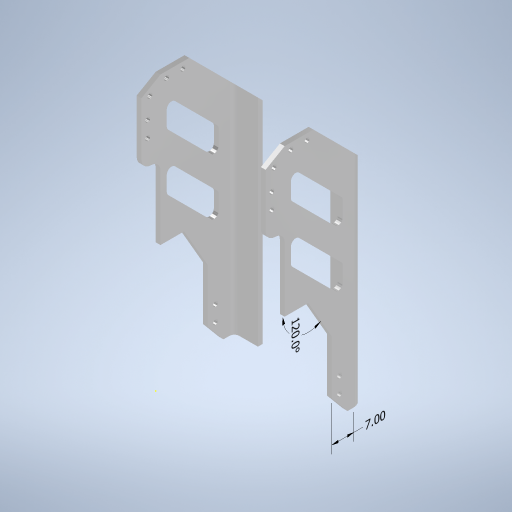
# Autodesk Inventor part: side
Saved by Autodesk Inventor 2024.1 (Build 281209000, 209)
## iProperties
Created: 2024-10-11
Part Number: side
Material: アルミニウム 6061
Document SubType Name: Sheet Metal
Designer: hibik
Density: 2.7 g/cm^3
Sheet Metal Rule: Default_mm
Appearance: アルミニウム - フラット
Author: hibik
Autodesk Inventor part; units mm, degrees
ref_plane "YZ Plane" through (0, 0, 0) normal (1, 0, 0) x (0, 1, 0)
ref_plane "XZ Plane" through (0, 0, 0) normal (0, 1, 0) x (-1, 0, 0)
ref_plane "XY Plane" through (0, 0, 0) normal (0, 0, 1) x (1, 0, 0)
sketch "スケッチ1" plane through (0, 0, 0) normal (1, 0, 0) x (0, 1, 0)
  line L0 (0, 0) -> (85, 0)
  line L1 (85, 0) -> (85, -20)
  line L2 (85, -20) -> (0, -20)
  line L3 (0, -20) -> (0, 0)
  circle A0 centre (0, -20) radius 1.6
  line L4 (-4, 0) -> (85, 0)
  line L5 (85, 0) -> (85, -25)
  line L6 (85, -25) -> (-4, -25)
  line L7 (-4, -25) -> (-4, 0)
  line L8 (-23, 0) -> (103, 0)
  line L9 (11, 0) -> (11, -15)
  line L10 (11, -15) -> (-0.9175, -25)
  line L11 (11, -15) -> (28.0096, -15)
  line L12 (28.0096, -15) -> (41, -7.5)
  line L13 (41, -7.5) -> (41, 0)
  circle A1 centre (0, -20) radius 5
  point P0 (4.9999, -20.0347)
  point P1 (0, -25)
  dimension "d0" = 85
  dimension "d1" = 20
  dimension "d2" = 3.2
  dimension "d3" = 4
  dimension "d4" = 5
  dimension "d5" = 5
  dimension "d6" = 11
  dimension "d7" = 50
  dimension "d8" = 7.5
  dimension "d9" = 120
  dimension "d10" = 41
  dimension "d11" = 15
  dimension "d12" = 10
  measures "d0" distance of L1.end L2.end
  measures "d1" distance of L2.end L0.start
  measures "d2" diameter of A0
  measures "d3" distance between parallel lines of L3 L7
  measures "d4" distance between parallel lines of L6 L2
  measures "d5" vertical distance of L9.end L2.end
  measures "d6" distance from line of L9 A0.centre
  measures "d7" angle of L9 L10
  measures "d8" distance of L12.end L13.end
  measures "d9" angle of L12 L13
  measures "d10" distance from line of L2.end L13
  measures "d11" distance between parallel lines of L0 L11
  measures "d12" diameter of A1
extrude "プレート1" add sketch "スケッチ1" along normal blind 1.5 contours L0 L1 L2 L10 L11 L12 L13 | L2 L5 L6 A1 L10
sketch "スケッチ2" plane through (1.5, 0, 0) normal (1, 0, 0) x (0, 0, -1)
  line L0 (2, 85) -> (2, 41)
  line L1 (0, 41) -> (0, 85) projected
  line L2 (7.5, 41) -> (0, 41) projected
  line L3 (0, 85) -> (25, 85) projected
  line L4 (2, 81) -> (18.5, 64.5)
  line L5 (18.5, 64.5) -> (18.5, 55.5)
  line L6 (18.5, 55.5) -> (2, 72)
  line L7 (2, 63) -> (18.5, 46.5)
  line L8 (18.5, 46.5) -> (18.5, 37.5)
  line L9 (18.5, 37.5) -> (2, 54)
  line L10 (25, 85) -> (25, 0) projected
  point P0 (0, 0)
  dimension "d14" = 2
  dimension "d15" = 135
  dimension "d16" = 9
  dimension "d17" = 6.5
  dimension "d18" = 9
  dimension "d19" = 13
  constraints: 14 end point, 5 point on line, 4 equal length, 2 collinear, 1 midpoint, 1 vertical
  measures "d14" distance between parallel lines of L1 L0
  measures "d15" angle of L0 L6
  measures "d16" distance of L4.end L5.end
  measures "d17" distance between parallel lines of L10 L5
  measures "d18" distance of L7.start L6.end
  measures "d19" distance from line of L2 L9.end
extrude "切り取り1" cut sketch "スケッチ2" against normal blind 1.5 contours L4 L5 L6 L0 | L7 L8 L9 L0
sketch "スケッチ3" plane through (1.5, 0, -23.5) normal (0, 0, -1) x (-1, 0, 0)
  line L0 (0, 85) -> (0, 0)
  line L1 (0, 0) -> (41, 0)
  line L2 (41, 0) -> (41, 85)
  line L3 (41, 85) -> (0, 85)
  constraints: 6 end point, 1 horizontal, 1 perpendicular, 1 vertical
edge flange "フランジ1" height 41 angle 90 thickness 1.5 bend radius 1.5 thickness toward (0, 0, -1) relief straight relief width 1.5 relief depth 0.75 edges at (0, 42.5, -25) wall of the first edge with corners at (1.5, 85, -23.5) (1.5, 0, -23.5) (-39.5, 0, -23.5) (-39.5, 85, -23.5)
bend "曲げ1"
corner "コーナー1"
sketch "スケッチ4" plane through (-38, 0, -25) normal (-1, 0, 0) x (0, -1, 0)
  line L0 (-85, 0) -> (0, 0)
  line L1 (0, 0) -> (0, 25)
  line L2 (0, 25) -> (-85, 25)
  line L3 (-85, 25) -> (-85, 0)
  constraints: 6 end point, 1 horizontal, 1 perpendicular, 1 vertical
edge flange "フランジ2" height 25 angle 90 thickness 1.5 bend radius 1.5 thickness toward (-1, 0, 0) relief straight relief width 1.5 relief depth 0.75 edges at (-39.5, 42.5, -23.5) wall of the first edge with corners at (-38, 85, -25) (-38, 0, -25) (-38, 0, 0) (-38, 85, 0)
bend "曲げ2"
corner "コーナー2"
sketch "スケッチ5" plane through (-38, 0, 0) normal (1, 0, 0) x (0, 0, -1)
  line L0 (22, 4.5826) -> (22, 85) projected
  line L1 (0, 85) -> (22, 85) projected
  line L2 (7.5, 41) -> (0, 41) projected
  line L3 (15, 28.0096) -> (7.5, 41) projected
  line L4 (15, 11) -> (15, 28.0096) projected
  line L5 (20.0347, 4.9999) -> (15, 11) projected
  arc A0 (22, 4.5826) -> (20.0347, 4.9999) centre (20, 0) ccw projected
  line L6 (18.5, 37.5) -> (2, 54) projected
  line L7 (2, 54) -> (2, 63) projected
  line L8 (2, 63) -> (18.5, 46.5) projected
  line L9 (18.5, 46.5) -> (18.5, 37.5) projected
  line L10 (2, 72) -> (2, 81) projected
  line L11 (22, 0) -> (22, 85) projected
  line L12 (22, 85) -> (0, 85) projected
  line L13 (0, 85) -> (0, 0) projected
  line L14 (22, 0) -> (0, 0) projected
  line L15 (2, 81) -> (18.5, 64.5) projected
  line L16 (18.5, 64.5) -> (18.5, 55.5) projected
  line L17 (18.5, 55.5) -> (2, 72) projected
  line L18 (0, 41) -> (0, 85) projected
  point P0 (0, 0)
  point P1 (0, 41)
  point P2 (22, 4.5826)
  point P3 (2, 85)
extrude "押し出し1" cut sketch "スケッチ5" against normal through all contours L11 L14 L13 L2 L3 L4 L5 A0 | L6 L7 L8 L9 | L10 L15 L16 L17
sketch "スケッチ7" plane through (-1.5, 0, -25) normal (0, 0, -1) x (-1, 0, 0)
  line L0 (0, 85) -> (35, 85) projected
  line L1 (6, 85) -> (29, 85)
  line L2 (29, 85) -> (29, 0)
  line L3 (29, 0) -> (6, 0)
  line L4 (6, 0) -> (6, 85)
  line L5 (0, 85) -> (0, 0) projected
  line L6 (35, 0) -> (35, 85) projected
  line L7 (6.1906, 67) -> (15.1906, 67) construction
  line L8 (15.1906, 67) -> (10.6906, 59.2058) construction
  line L9 (10.6906, 59.2058) -> (6.1906, 67) construction
  arc A0 (8.7887, 67) -> (7.4896, 64.75) centre (8.7887, 65.5) ccw
  arc A1 (13.8916, 64.75) -> (12.5925, 67) centre (12.5925, 65.5) ccw
  arc A2 (9.3916, 61.4558) -> (11.9896, 61.4558) centre (10.6906, 62.2058) ccw
  line L10 (17.5, 67) -> (13, 59.2058) construction
  line L11 (13, 59.2058) -> (22, 59.2058) construction
  line L12 (22, 59.2058) -> (17.5, 67) construction
  arc A3 (18.799, 64.75) -> (16.201, 64.75) centre (17.5, 64) ccw
  arc A4 (14.299, 61.4558) -> (15.5981, 59.2058) centre (15.5981, 60.7058) ccw
  arc A5 (19.4019, 59.2058) -> (20.701, 61.4558) centre (19.4019, 60.7058) ccw
  line L13 (8.7887, 67) -> (12.5925, 67)
  line L14 (13.8916, 64.75) -> (11.9896, 61.4558)
  line L15 (7.4896, 64.75) -> (9.3916, 61.4558)
  line L16 (16.201, 64.75) -> (14.299, 61.4558)
  line L17 (15.5981, 59.2058) -> (19.4019, 59.2058)
  line L18 (20.701, 61.4558) -> (18.799, 64.75)
  line L19 (19.8094, 67) -> (28.8094, 67) construction
  line L20 (28.8094, 67) -> (24.3094, 59.2058) construction
  line L21 (24.3094, 59.2058) -> (19.8094, 67) construction
  arc A6 (22.4075, 67) -> (21.1084, 64.75) centre (22.4075, 65.5) ccw
  arc A7 (27.5104, 64.75) -> (26.2113, 67) centre (26.2113, 65.5) ccw
  arc A8 (23.0104, 61.4558) -> (25.6084, 61.4558) centre (24.3094, 62.2058) ccw
  line L22 (22.4075, 67) -> (26.2113, 67)
  line L23 (27.5104, 64.75) -> (25.6084, 61.4558)
  line L24 (21.1084, 64.75) -> (23.0104, 61.4558)
  line L25 (6, 58.2058) -> (29, 58.2058) construction
  line L26 (6.1906, 49.4115) -> (15.1906, 49.4115) construction
  line L27 (15.1906, 49.4115) -> (10.6906, 57.2058) construction
  line L28 (10.6906, 57.2058) -> (6.1906, 49.4115) construction
  arc A9 (7.4896, 51.6615) -> (8.7887, 49.4115) centre (8.7887, 50.9115) ccw
  arc A10 (12.5925, 49.4115) -> (13.8916, 51.6615) centre (12.5925, 50.9115) ccw
  arc A11 (11.9896, 54.9558) -> (9.3916, 54.9558) centre (10.6906, 54.2058) ccw
  line L29 (17.5, 49.4115) -> (13, 57.2058) construction
  line L30 (13, 57.2058) -> (22, 57.2058) construction
  line L31 (22, 57.2058) -> (17.5, 49.4115) construction
  arc A12 (16.201, 51.6615) -> (18.799, 51.6615) centre (17.5, 52.4115) ccw
  arc A13 (15.5981, 57.2058) -> (14.299, 54.9558) centre (15.5981, 55.7058) ccw
  arc A14 (20.701, 54.9558) -> (19.4019, 57.2058) centre (19.4019, 55.7058) ccw
  line L32 (8.7887, 49.4115) -> (12.5925, 49.4115)
  line L33 (13.8916, 51.6615) -> (11.9896, 54.9558)
  line L34 (7.4896, 51.6615) -> (9.3916, 54.9558)
  line L35 (16.201, 51.6615) -> (14.299, 54.9558)
  line L36 (15.5981, 57.2058) -> (19.4019, 57.2058)
  line L37 (20.701, 54.9558) -> (18.799, 51.6615)
  line L38 (19.8094, 49.4115) -> (28.8094, 49.4115) construction
  line L39 (28.8094, 49.4115) -> (24.3094, 57.2058) construction
  line L40 (24.3094, 57.2058) -> (19.8094, 49.4115) construction
  arc A15 (21.1084, 51.6615) -> (22.4075, 49.4115) centre (22.4075, 50.9115) ccw
  arc A16 (26.2113, 49.4115) -> (27.5104, 51.6615) centre (26.2113, 50.9115) ccw
  line L41 (27.5104, 51.6615) -> (25.6084, 54.9558)
  arc A17 (25.6084, 54.9558) -> (23.0104, 54.9558) centre (24.3094, 54.2058) ccw
  line L42 (22.4075, 49.4115) -> (26.2113, 49.4115)
  line L43 (21.1084, 51.6615) -> (23.0104, 54.9558)
  arc A18 (5.1802, 64.75) -> (2.5822, 64.75) centre (3.8812, 64) ccw
  arc A19 (5.7831, 59.2058) -> (7.0822, 61.4558) centre (5.7831, 60.7058) ccw
  line L44 (7.0822, 61.4558) -> (5.1802, 64.75)
  line L45 (5.7831, 59.2058) -> (-10.927, 59.2058)
  arc A20 (32.4178, 64.75) -> (29.8198, 64.75) centre (31.1188, 64) ccw
  arc A21 (27.9178, 61.4558) -> (29.2169, 59.2058) centre (29.2169, 60.7058) ccw
  line L46 (29.8198, 64.75) -> (27.9178, 61.4558)
  line L47 (29.2169, 59.2058) -> (29, 59.2058)
  line L48 (7.0822, 54.9558) -> (5.1802, 51.6615)
  arc A22 (2.5822, 51.6615) -> (5.1802, 51.6615) centre (3.8812, 52.4115) ccw
  arc A23 (7.0822, 54.9558) -> (5.7831, 57.2058) centre (5.7831, 55.7058) ccw
  line L49 (5.7831, 57.2058) -> (-10.927, 57.2058)
  line L50 (29.8198, 51.6615) -> (27.9178, 54.9558)
  arc A24 (29.8198, 51.6615) -> (32.4178, 51.6615) centre (31.1188, 52.4115) ccw
  arc A25 (29.2169, 57.2058) -> (27.9178, 54.9558) centre (29.2169, 55.7058) ccw
  line L51 (29.2169, 57.2058) -> (29, 57.2058)
  line L52 (6.1906, 47.4115) -> (15.1906, 47.4115) construction
  line L53 (15.1906, 47.4115) -> (10.6906, 39.6173) construction
  arc A26 (9.3916, 41.8673) -> (11.9896, 41.8673) centre (10.6906, 42.6173) ccw
  line L54 (8.7887, 47.4115) -> (12.5925, 47.4115)
  line L55 (13.8916, 45.1615) -> (11.9896, 41.8673)
  arc A27 (13.8916, 45.1615) -> (12.5925, 47.4115) centre (12.5925, 45.9115) ccw
  arc A28 (14.299, 41.8673) -> (15.5981, 39.6173) centre (15.5981, 41.1173) ccw
  line L56 (16.201, 45.1615) -> (14.299, 41.8673)
  arc A29 (18.799, 45.1615) -> (16.201, 45.1615) centre (17.5, 44.4115) ccw
  line L57 (17.5, 47.4115) -> (13, 39.6173) construction
  arc A30 (27.9178, 41.8673) -> (29.2169, 39.6173) centre (29.2169, 41.1173) ccw
  line L58 (29.8198, 45.1615) -> (27.9178, 41.8673)
  arc A31 (32.4178, 45.1615) -> (29.8198, 45.1615) centre (31.1188, 44.4115) ccw
  line L59 (29.2169, 39.6173) -> (29, 39.6173)
  line L60 (22, 39.6173) -> (17.5, 47.4115) construction
  arc A32 (19.4019, 39.6173) -> (20.701, 41.8673) centre (19.4019, 41.1173) ccw
  line L61 (27.5104, 45.1615) -> (25.6084, 41.8673)
  arc A33 (23.0104, 41.8673) -> (25.6084, 41.8673) centre (24.3094, 42.6173) ccw
  arc A34 (27.5104, 45.1615) -> (26.2113, 47.4115) centre (26.2113, 45.9115) ccw
  line L62 (28.8094, 47.4115) -> (24.3094, 39.6173) construction
  line L63 (22.4075, 47.4115) -> (26.2113, 47.4115)
  line L64 (19.8094, 47.4115) -> (28.8094, 47.4115) construction
  line L65 (21.1084, 45.1615) -> (23.0104, 41.8673)
  line L66 (24.3094, 39.6173) -> (19.8094, 47.4115) construction
  line L67 (20.701, 41.8673) -> (18.799, 45.1615)
  arc A35 (22.4075, 47.4115) -> (21.1084, 45.1615) centre (22.4075, 45.9115) ccw
  arc A36 (20.701, 35.3673) -> (19.4019, 37.6173) centre (19.4019, 36.1173) ccw
  line L68 (20.701, 35.3673) -> (18.799, 32.0731)
  line L69 (22, 37.6173) -> (17.5, 29.8231) construction
  arc A37 (16.201, 32.0731) -> (18.799, 32.0731) centre (17.5, 32.8231) ccw
  line L70 (15.5981, 37.6173) -> (19.4019, 37.6173)
  line L71 (13, 37.6173) -> (22, 37.6173) construction
  line L72 (16.201, 32.0731) -> (14.299, 35.3673)
  line L73 (17.5, 29.8231) -> (13, 37.6173) construction
  arc A38 (15.5981, 37.6173) -> (14.299, 35.3673) centre (15.5981, 36.1173) ccw
  line L74 (6.1906, 29.8231) -> (15.1906, 29.8231) construction
  line L75 (15.1906, 29.8231) -> (10.6906, 37.6173) construction
  line L76 (10.6906, 37.6173) -> (6.1906, 29.8231) construction
  arc A39 (7.4896, 32.0731) -> (8.7887, 29.8231) centre (8.7887, 31.3231) ccw
  line L77 (5.7831, 37.6173) -> (-10.927, 37.6173)
  arc A40 (7.0822, 35.3673) -> (5.7831, 37.6173) centre (5.7831, 36.1173) ccw
  arc A41 (2.5822, 32.0731) -> (5.1802, 32.0731) centre (3.8812, 32.8231) ccw
  line L78 (7.0822, 35.3673) -> (5.1802, 32.0731)
  arc A42 (11.9896, 35.3673) -> (9.3916, 35.3673) centre (10.6906, 34.6173) ccw
  line L79 (7.4896, 32.0731) -> (9.3916, 35.3673)
  line L80 (13.8916, 32.0731) -> (11.9896, 35.3673)
  line L81 (8.7887, 29.8231) -> (12.5925, 29.8231)
  arc A43 (12.5925, 29.8231) -> (13.8916, 32.0731) centre (12.5925, 31.3231) ccw
  line L82 (13, 39.6173) -> (22, 39.6173) construction
  line L83 (15.5981, 39.6173) -> (19.4019, 39.6173)
  line L84 (6, 38.6173) -> (29, 38.6173) construction
  line L85 (27.5104, 32.0731) -> (25.6084, 35.3673)
  line L86 (28.8094, 29.8231) -> (24.3094, 37.6173) construction
  arc A44 (26.2113, 29.8231) -> (27.5104, 32.0731) centre (26.2113, 31.3231) ccw
  arc A45 (25.6084, 35.3673) -> (23.0104, 35.3673) centre (24.3094, 34.6173) ccw
  line L87 (21.1084, 32.0731) -> (23.0104, 35.3673)
  arc A46 (21.1084, 32.0731) -> (22.4075, 29.8231) centre (22.4075, 31.3231) ccw
  line L88 (24.3094, 37.6173) -> (19.8094, 29.8231) construction
  line L89 (22.4075, 29.8231) -> (26.2113, 29.8231)
  arc A47 (29.2169, 37.6173) -> (27.9178, 35.3673) centre (29.2169, 36.1173) ccw
  line L90 (19.8094, 29.8231) -> (28.8094, 29.8231) construction
  line L91 (29.8198, 32.0731) -> (27.9178, 35.3673)
  line L92 (29.2169, 37.6173) -> (29, 37.6173)
  arc A48 (29.8198, 32.0731) -> (32.4178, 32.0731) centre (31.1188, 32.8231) ccw
  line L93 (10.6906, 39.6173) -> (6.1906, 47.4115) construction
  arc A49 (8.7887, 47.4115) -> (7.4896, 45.1615) centre (8.7887, 45.9115) ccw
  line L94 (7.4896, 45.1615) -> (9.3916, 41.8673)
  arc A50 (5.7831, 39.6173) -> (7.0822, 41.8673) centre (5.7831, 41.1173) ccw
  line L95 (7.0822, 41.8673) -> (5.1802, 45.1615)
  arc A51 (5.1802, 45.1615) -> (2.5822, 45.1615) centre (3.8812, 44.4115) ccw
  line L96 (5.7831, 39.6173) -> (-10.927, 39.6173)
  line L97 (6.1906, 27.8231) -> (15.1906, 27.8231) construction
  line L98 (15.1906, 27.8231) -> (10.6906, 20.0289) construction
  arc A52 (9.3916, 22.2789) -> (11.9896, 22.2789) centre (10.6906, 23.0289) ccw
  line L99 (8.7887, 27.8231) -> (12.5925, 27.8231)
  line L100 (13.8916, 25.5731) -> (11.9896, 22.2789)
  arc A53 (13.8916, 25.5731) -> (12.5925, 27.8231) centre (12.5925, 26.3231) ccw
  arc A54 (14.299, 22.2789) -> (15.5981, 20.0289) centre (15.5981, 21.5289) ccw
  line L101 (16.201, 25.5731) -> (14.299, 22.2789)
  arc A55 (18.799, 25.5731) -> (16.201, 25.5731) centre (17.5, 24.8231) ccw
  line L102 (17.5, 27.8231) -> (13, 20.0289) construction
  arc A56 (27.9178, 22.2789) -> (29.2169, 20.0289) centre (29.2169, 21.5289) ccw
  line L103 (29.8198, 25.5731) -> (27.9178, 22.2789)
  arc A57 (32.4178, 25.5731) -> (29.8198, 25.5731) centre (31.1188, 24.8231) ccw
  line L104 (29.2169, 20.0289) -> (29, 20.0289)
  line L105 (22, 20.0289) -> (17.5, 27.8231) construction
  arc A58 (19.4019, 20.0289) -> (20.701, 22.2789) centre (19.4019, 21.5289) ccw
  line L106 (27.5104, 25.5731) -> (25.6084, 22.2789)
  arc A59 (23.0104, 22.2789) -> (25.6084, 22.2789) centre (24.3094, 23.0289) ccw
  arc A60 (27.5104, 25.5731) -> (26.2113, 27.8231) centre (26.2113, 26.3231) ccw
  line L107 (28.8094, 27.8231) -> (24.3094, 20.0289) construction
  line L108 (22.4075, 27.8231) -> (26.2113, 27.8231)
  line L109 (19.8094, 27.8231) -> (28.8094, 27.8231) construction
  line L110 (21.1084, 25.5731) -> (23.0104, 22.2789)
  line L111 (24.3094, 20.0289) -> (19.8094, 27.8231) construction
  line L112 (20.701, 22.2789) -> (18.799, 25.5731)
  arc A61 (22.4075, 27.8231) -> (21.1084, 25.5731) centre (22.4075, 26.3231) ccw
  arc A62 (20.701, 15.7789) -> (19.4019, 18.0289) centre (19.4019, 16.5289) ccw
  line L113 (20.701, 15.7789) -> (18.799, 12.4846)
  line L114 (22, 18.0289) -> (17.5, 10.2346) construction
  arc A63 (16.201, 12.4846) -> (18.799, 12.4846) centre (17.5, 13.2346) ccw
  line L115 (15.5981, 18.0289) -> (19.4019, 18.0289)
  line L116 (13, 18.0289) -> (22, 18.0289) construction
  line L117 (16.201, 12.4846) -> (14.299, 15.7789)
  line L118 (17.5, 10.2346) -> (13, 18.0289) construction
  arc A64 (15.5981, 18.0289) -> (14.299, 15.7789) centre (15.5981, 16.5289) ccw
  line L119 (6.1906, 10.2346) -> (15.1906, 10.2346) construction
  line L120 (15.1906, 10.2346) -> (10.6906, 18.0289) construction
  line L121 (10.6906, 18.0289) -> (6.1906, 10.2346) construction
  arc A65 (7.4896, 12.4846) -> (8.7887, 10.2346) centre (8.7887, 11.7346) ccw
  line L122 (5.7831, 18.0289) -> (-10.927, 18.0289)
  arc A66 (7.0822, 15.7789) -> (5.7831, 18.0289) centre (5.7831, 16.5289) ccw
  arc A67 (2.5822, 12.4846) -> (5.1802, 12.4846) centre (3.8812, 13.2346) ccw
  line L123 (7.0822, 15.7789) -> (5.1802, 12.4846)
  arc A68 (11.9896, 15.7789) -> (9.3916, 15.7789) centre (10.6906, 15.0289) ccw
  line L124 (7.4896, 12.4846) -> (9.3916, 15.7789)
  line L125 (13.8916, 12.4846) -> (11.9896, 15.7789)
  line L126 (8.7887, 10.2346) -> (12.5925, 10.2346)
  arc A69 (12.5925, 10.2346) -> (13.8916, 12.4846) centre (12.5925, 11.7346) ccw
  line L127 (13, 20.0289) -> (22, 20.0289) construction
  line L128 (15.5981, 20.0289) -> (19.4019, 20.0289)
  line L129 (6, 19.0289) -> (29, 19.0289) construction
  line L130 (27.5104, 12.4846) -> (25.6084, 15.7789)
  line L131 (28.8094, 10.2346) -> (24.3094, 18.0289) construction
  arc A70 (26.2113, 10.2346) -> (27.5104, 12.4846) centre (26.2113, 11.7346) ccw
  arc A71 (25.6084, 15.7789) -> (23.0104, 15.7789) centre (24.3094, 15.0289) ccw
  line L132 (21.1084, 12.4846) -> (23.0104, 15.7789)
  arc A72 (21.1084, 12.4846) -> (22.4075, 10.2346) centre (22.4075, 11.7346) ccw
  line L133 (24.3094, 18.0289) -> (19.8094, 10.2346) construction
  line L134 (22.4075, 10.2346) -> (26.2113, 10.2346)
  arc A73 (29.2169, 18.0289) -> (27.9178, 15.7789) centre (29.2169, 16.5289) ccw
  line L135 (19.8094, 10.2346) -> (28.8094, 10.2346) construction
  line L136 (29.8198, 12.4846) -> (27.9178, 15.7789)
  line L137 (29.2169, 18.0289) -> (29, 18.0289)
  arc A74 (29.8198, 12.4846) -> (32.4178, 12.4846) centre (31.1188, 13.2346) ccw
  line L138 (10.6906, 20.0289) -> (6.1906, 27.8231) construction
  arc A75 (8.7887, 27.8231) -> (7.4896, 25.5731) centre (8.7887, 26.3231) ccw
  line L139 (7.4896, 25.5731) -> (9.3916, 22.2789)
  arc A76 (5.7831, 20.0289) -> (7.0822, 22.2789) centre (5.7831, 21.5289) ccw
  line L140 (7.0822, 22.2789) -> (5.1802, 25.5731)
  arc A77 (5.1802, 25.5731) -> (2.5822, 25.5731) centre (3.8812, 24.8231) ccw
  line L141 (5.7831, 20.0289) -> (-10.927, 20.0289)
  line L142 (6.1906, 8.2346) -> (15.1906, 8.2346) construction
  line L143 (15.1906, 8.2346) -> (10.6906, 0.4404) construction
  arc A78 (9.3916, 2.6904) -> (11.9896, 2.6904) centre (10.6906, 3.4404) ccw
  line L144 (8.7887, 8.2346) -> (12.5925, 8.2346)
  line L145 (13.8916, 5.9846) -> (11.9896, 2.6904)
  arc A79 (13.8916, 5.9846) -> (12.5925, 8.2346) centre (12.5925, 6.7346) ccw
  arc A80 (14.299, 2.6904) -> (15.5981, 0.4404) centre (15.5981, 1.9404) ccw
  line L146 (16.201, 5.9846) -> (14.299, 2.6904)
  arc A81 (18.799, 5.9846) -> (16.201, 5.9846) centre (17.5, 5.2346) ccw
  line L147 (17.5, 8.2346) -> (13, 0.4404) construction
  arc A82 (27.9178, 2.6904) -> (29.2169, 0.4404) centre (29.2169, 1.9404) ccw
  line L148 (29.8198, 5.9846) -> (27.9178, 2.6904)
  arc A83 (32.4178, 5.9846) -> (29.8198, 5.9846) centre (31.1188, 5.2346) ccw
  line L149 (29.2169, 0.4404) -> (29, 0.4404)
  line L150 (22, 0.4404) -> (17.5, 8.2346) construction
  arc A84 (19.4019, 0.4404) -> (20.701, 2.6904) centre (19.4019, 1.9404) ccw
  line L151 (27.5104, 5.9846) -> (25.6084, 2.6904)
  arc A85 (23.0104, 2.6904) -> (25.6084, 2.6904) centre (24.3094, 3.4404) ccw
  arc A86 (27.5104, 5.9846) -> (26.2113, 8.2346) centre (26.2113, 6.7346) ccw
  line L152 (28.8094, 8.2346) -> (24.3094, 0.4404) construction
  line L153 (22.4075, 8.2346) -> (26.2113, 8.2346)
  line L154 (19.8094, 8.2346) -> (28.8094, 8.2346) construction
  line L155 (21.1084, 5.9846) -> (23.0104, 2.6904)
  line L156 (24.3094, 0.4404) -> (19.8094, 8.2346) construction
  line L157 (20.701, 2.6904) -> (18.799, 5.9846)
  arc A87 (22.4075, 8.2346) -> (21.1084, 5.9846) centre (22.4075, 6.7346) ccw
  arc A88 (20.701, -3.8096) -> (19.4019, -1.5596) centre (19.4019, -3.0596) ccw
  line L158 (20.701, -3.8096) -> (18.799, -7.1038)
  line L159 (22, -1.5596) -> (17.5, -9.3538) construction
  arc A89 (16.201, -7.1038) -> (18.799, -7.1038) centre (17.5, -6.3538) ccw
  line L160 (15.5981, -1.5596) -> (19.4019, -1.5596)
  line L161 (13, -1.5596) -> (22, -1.5596) construction
  line L162 (16.201, -7.1038) -> (14.299, -3.8096)
  line L163 (17.5, -9.3538) -> (13, -1.5596) construction
  arc A90 (15.5981, -1.5596) -> (14.299, -3.8096) centre (15.5981, -3.0596) ccw
  line L164 (6.1906, -9.3538) -> (15.1906, -9.3538) construction
  line L165 (15.1906, -9.3538) -> (10.6906, -1.5596) construction
  line L166 (10.6906, -1.5596) -> (6.1906, -9.3538) construction
  arc A91 (7.4896, -7.1038) -> (8.7887, -9.3538) centre (8.7887, -7.8538) ccw
  line L167 (5.7831, -1.5596) -> (-10.927, -1.5596)
  arc A92 (7.0822, -3.8096) -> (5.7831, -1.5596) centre (5.7831, -3.0596) ccw
  arc A93 (2.5822, -7.1038) -> (5.1802, -7.1038) centre (3.8812, -6.3538) ccw
  line L168 (7.0822, -3.8096) -> (5.1802, -7.1038)
  arc A94 (11.9896, -3.8096) -> (9.3916, -3.8096) centre (10.6906, -4.5596) ccw
  line L169 (7.4896, -7.1038) -> (9.3916, -3.8096)
  line L170 (13.8916, -7.1038) -> (11.9896, -3.8096)
  line L171 (8.7887, -9.3538) -> (12.5925, -9.3538)
  arc A95 (12.5925, -9.3538) -> (13.8916, -7.1038) centre (12.5925, -7.8538) ccw
  line L172 (13, 0.4404) -> (22, 0.4404) construction
  line L173 (15.5981, 0.4404) -> (19.4019, 0.4404)
  line L174 (6, -0.5596) -> (29, -0.5596) construction
  line L175 (27.5104, -7.1038) -> (25.6084, -3.8096)
  line L176 (28.8094, -9.3538) -> (24.3094, -1.5596) construction
  arc A96 (26.2113, -9.3538) -> (27.5104, -7.1038) centre (26.2113, -7.8538) ccw
  arc A97 (25.6084, -3.8096) -> (23.0104, -3.8096) centre (24.3094, -4.5596) ccw
  line L177 (21.1084, -7.1038) -> (23.0104, -3.8096)
  arc A98 (21.1084, -7.1038) -> (22.4075, -9.3538) centre (22.4075, -7.8538) ccw
  line L178 (24.3094, -1.5596) -> (19.8094, -9.3538) construction
  line L179 (22.4075, -9.3538) -> (26.2113, -9.3538)
  arc A99 (29.2169, -1.5596) -> (27.9178, -3.8096) centre (29.2169, -3.0596) ccw
  line L180 (19.8094, -9.3538) -> (28.8094, -9.3538) construction
  line L181 (29.8198, -7.1038) -> (27.9178, -3.8096)
  line L182 (29.2169, -1.5596) -> (29, -1.5596)
  arc A100 (29.8198, -7.1038) -> (32.4178, -7.1038) centre (31.1188, -6.3538) ccw
  line L183 (10.6906, 0.4404) -> (6.1906, 8.2346) construction
  arc A101 (8.7887, 8.2346) -> (7.4896, 5.9846) centre (8.7887, 6.7346) ccw
  line L184 (7.4896, 5.9846) -> (9.3916, 2.6904)
  arc A102 (5.7831, 0.4404) -> (7.0822, 2.6904) centre (5.7831, 1.9404) ccw
  line L185 (7.0822, 2.6904) -> (5.1802, 5.9846)
  arc A103 (5.1802, 5.9846) -> (2.5822, 5.9846) centre (3.8812, 5.2346) ccw
  line L186 (5.7831, 0.4404) -> (-10.927, 0.4404)
  line L187 (6.1906, -11.3538) -> (15.1906, -11.3538) construction
  line L188 (15.1906, -11.3538) -> (10.6906, -19.1481) construction
  arc A104 (9.3916, -16.8981) -> (11.9896, -16.8981) centre (10.6906, -16.1481) ccw
  line L189 (8.7887, -11.3538) -> (12.5925, -11.3538)
  line L190 (13.8916, -13.6038) -> (11.9896, -16.8981)
  arc A105 (13.8916, -13.6038) -> (12.5925, -11.3538) centre (12.5925, -12.8538) ccw
  arc A106 (14.299, -16.8981) -> (15.5981, -19.1481) centre (15.5981, -17.6481) ccw
  line L191 (16.201, -13.6038) -> (14.299, -16.8981)
  arc A107 (18.799, -13.6038) -> (16.201, -13.6038) centre (17.5, -14.3538) ccw
  line L192 (17.5, -11.3538) -> (13, -19.1481) construction
  arc A108 (27.9178, -16.8981) -> (29.2169, -19.1481) centre (29.2169, -17.6481) ccw
  line L193 (29.8198, -13.6038) -> (27.9178, -16.8981)
  arc A109 (32.4178, -13.6038) -> (29.8198, -13.6038) centre (31.1188, -14.3538) ccw
  line L194 (29.2169, -19.1481) -> (29, -19.1481)
  line L195 (22, -19.1481) -> (17.5, -11.3538) construction
  arc A110 (19.4019, -19.1481) -> (20.701, -16.8981) centre (19.4019, -17.6481) ccw
  line L196 (27.5104, -13.6038) -> (25.6084, -16.8981)
  arc A111 (23.0104, -16.8981) -> (25.6084, -16.8981) centre (24.3094, -16.1481) ccw
  arc A112 (27.5104, -13.6038) -> (26.2113, -11.3538) centre (26.2113, -12.8538) ccw
  line L197 (28.8094, -11.3538) -> (24.3094, -19.1481) construction
  line L198 (22.4075, -11.3538) -> (26.2113, -11.3538)
  line L199 (19.8094, -11.3538) -> (28.8094, -11.3538) construction
  line L200 (21.1084, -13.6038) -> (23.0104, -16.8981)
  line L201 (24.3094, -19.1481) -> (19.8094, -11.3538) construction
  line L202 (20.701, -16.8981) -> (18.799, -13.6038)
  arc A113 (22.4075, -11.3538) -> (21.1084, -13.6038) centre (22.4075, -12.8538) ccw
  arc A114 (20.701, -23.3981) -> (19.4019, -21.1481) centre (19.4019, -22.6481) ccw
  line L203 (20.701, -23.3981) -> (18.799, -26.6923)
  line L204 (22, -21.1481) -> (17.5, -28.9423) construction
  arc A115 (16.201, -26.6923) -> (18.799, -26.6923) centre (17.5, -25.9423) ccw
  line L205 (15.5981, -21.1481) -> (19.4019, -21.1481)
  line L206 (13, -21.1481) -> (22, -21.1481) construction
  line L207 (16.201, -26.6923) -> (14.299, -23.3981)
  line L208 (17.5, -28.9423) -> (13, -21.1481) construction
  arc A116 (15.5981, -21.1481) -> (14.299, -23.3981) centre (15.5981, -22.6481) ccw
  line L209 (6.1906, -28.9423) -> (15.1906, -28.9423) construction
  line L210 (15.1906, -28.9423) -> (10.6906, -21.1481) construction
  line L211 (10.6906, -21.1481) -> (6.1906, -28.9423) construction
  arc A117 (7.4896, -26.6923) -> (8.7887, -28.9423) centre (8.7887, -27.4423) ccw
  line L212 (5.7831, -21.1481) -> (-10.927, -21.1481)
  arc A118 (7.0822, -23.3981) -> (5.7831, -21.1481) centre (5.7831, -22.6481) ccw
  arc A119 (2.5822, -26.6923) -> (5.1802, -26.6923) centre (3.8812, -25.9423) ccw
  line L213 (7.0822, -23.3981) -> (5.1802, -26.6923)
  arc A120 (11.9896, -23.3981) -> (9.3916, -23.3981) centre (10.6906, -24.1481) ccw
  line L214 (7.4896, -26.6923) -> (9.3916, -23.3981)
  line L215 (13.8916, -26.6923) -> (11.9896, -23.3981)
  line L216 (8.7887, -28.9423) -> (12.5925, -28.9423)
  arc A121 (12.5925, -28.9423) -> (13.8916, -26.6923) centre (12.5925, -27.4423) ccw
  line L217 (13, -19.1481) -> (22, -19.1481) construction
  line L218 (15.5981, -19.1481) -> (19.4019, -19.1481)
  line L219 (6, -20.1481) -> (29, -20.1481) construction
  line L220 (27.5104, -26.6923) -> (25.6084, -23.3981)
  line L221 (28.8094, -28.9423) -> (24.3094, -21.1481) construction
  arc A122 (26.2113, -28.9423) -> (27.5104, -26.6923) centre (26.2113, -27.4423) ccw
  arc A123 (25.6084, -23.3981) -> (23.0104, -23.3981) centre (24.3094, -24.1481) ccw
  line L222 (21.1084, -26.6923) -> (23.0104, -23.3981)
  arc A124 (21.1084, -26.6923) -> (22.4075, -28.9423) centre (22.4075, -27.4423) ccw
  line L223 (24.3094, -21.1481) -> (19.8094, -28.9423) construction
  line L224 (22.4075, -28.9423) -> (26.2113, -28.9423)
  arc A125 (29.2169, -21.1481) -> (27.9178, -23.3981) centre (29.2169, -22.6481) ccw
  line L225 (19.8094, -28.9423) -> (28.8094, -28.9423) construction
  line L226 (29.8198, -26.6923) -> (27.9178, -23.3981)
  line L227 (29.2169, -21.1481) -> (29, -21.1481)
  arc A126 (29.8198, -26.6923) -> (32.4178, -26.6923) centre (31.1188, -25.9423) ccw
  line L228 (10.6906, -19.1481) -> (6.1906, -11.3538) construction
  arc A127 (8.7887, -11.3538) -> (7.4896, -13.6038) centre (8.7887, -12.8538) ccw
  line L229 (7.4896, -13.6038) -> (9.3916, -16.8981)
  arc A128 (5.7831, -19.1481) -> (7.0822, -16.8981) centre (5.7831, -17.6481) ccw
  line L230 (7.0822, -16.8981) -> (5.1802, -13.6038)
  arc A129 (5.1802, -13.6038) -> (2.5822, -13.6038) centre (3.8812, -14.3538) ccw
  line L231 (5.7831, -19.1481) -> (-10.927, -19.1481)
  line L232 (5.1802, 5.9846) -> (7.0822, 2.6904)
  arc A130 (6, 0.4562) -> (7.0822, 2.6904) centre (5.7831, 1.9404) ccw
  line L233 (5.7831, 0.4404) -> (4.7831, 0.4404)
  point P0 (-1.5, 0)
  point P1 (17.5, 85)
  point P2 (17.5, 65.4115)
  point P3 (6, 65.4115)
  point P4 (29, 65.4115)
  point P5 (17.5, 45.8231)
  point P6 (6, 45.8231)
  point P7 (29, 45.8231)
  point P8 (17.5, 26.2346)
  point P9 (6, 26.2346)
  point P10 (29, 26.2346)
  point P11 (17.5, 6.6462)
  point P12 (6, 6.6462)
  point P13 (29, 6.6462)
  point P14 (27.0333, 0)
  point P15 (22.5855, 0)
  point P16 (13.4145, 0)
  point P17 (8.9667, 0)
  point P18 (6, 12.1415)
  point P19 (6, 5.8519)
  point P20 (33, 17.1509)
  point P21 (30, 1.4404)
  point P22 (30, 5.8519)
  point P23 (33, 12.1415)
  point P24 (6, 31.7299)
  point P25 (6, 0.4404)
  point P26 (6, 1.4404)
  point P27 (6, 17.1509)
  point P28 (33, 36.7393)
  point P29 (33, 31.7299)
  point P30 (6, 18.0289)
  point P31 (6, 36.7393)
  point P32 (20.2761, 0)
  point P33 (15.7239, 0)
  point P34 (6, 51.3184)
  point P35 (6, 20.0289)
  point P36 (33, 56.3278)
  point P37 (29, 37.6173)
  point P38 (33, 51.3184)
  point P39 (6, 70.9068)
  point P40 (6, 39.6173)
  point P41 (6, 37.6173)
  point P42 (6, 56.3278)
  point P43 (6, 57.2058)
  point P44 (6, 75.9163)
  point P45 (29, 39.6173)
  point P46 (33, 70.9068)
  point P47 (33, 75.9163)
  point P48 (29, 57.2058)
  point P49 (30, 65.2058)
  point P50 (33, 90.4953)
  point P51 (6, 90.4953)
  point P52 (6, 59.2058)
  point P53 (6, 0.8423)
  point P54 (30, 8.45)
  point P55 (30, 0.8423)
  point P56 (6, 4.5648)
  point P57 (6, 8.45)
  point P58 (29, 13.9045)
  point P59 (29, 4.5648)
  point P60 (6, 13.9045)
  point P61 (6, 24.1532)
  point P62 (29, 33.493)
  point P63 (29, 24.1532)
  point P64 (6, 43.7417)
  point P65 (6, 33.493)
  point P66 (6, 53.0814)
  point P67 (29, 43.7417)
  point P68 (29, 53.0814)
  point P69 (29, 63.3301)
  point P70 (6, 63.3301)
  point P71 (29.5137, 0)
  point P72 (6.4863, 0)
  point P73 (27.2043, 0)
  point P74 (22.4145, 0)
  point P75 (20.1051, 0)
  point P76 (15.8949, 0)
  point P77 (13.5855, 0)
  point P78 (8.7957, 0)
  point P79 (6, 0.4562)
  point P80 (6.3175, 0)
  point P81 (19.9363, 0)
  point P82 (16.0637, 0)
  point P83 (27.3731, 0)
  point P84 (22.2457, 0)
  point P85 (13.7543, 0)
  point P86 (8.6269, 0)
  point P87 (21.4007, 0)
  point P88 (14.5993, 0)
  point P89 (6.2831, 0.4404)
  point P90 (6, 59.2215)
  point P91 (6, 20.0446)
  point P92 (6, 18.0131)
  point P93 (6, 39.6331)
  point P94 (6, 37.6016)
  point P95 (6, 57.19)
  point P96 (29, 18.0131)
  point P97 (29, 20.0446)
  point P98 (29, 37.6016)
  point P99 (29, 39.6331)
  point P100 (29, 57.19)
  point P101 (29, 59.2215)
  point P102 (6, 4.5648)
  dimension "d44" = 6
  dimension "d45" = 6
  dimension "d46" = 9
  dimension "d47" = 3
  dimension "d52" = 2
  dimension "d53" = 18
  dimension "d54" = 9
  dimension "d55" = 3
  dimension "d56" = 2
  dimension "d60" = 1
  dimension "d70" = 2
  dimension "d71" = 2
  dimension "d74" = 19.5885
  constraints: 456 end point, 421 vertical alignment, 263 point on circle, 212 point on line, 181 parallel, 131 centre point, 115 equal radius, 50 symmetric about line, 28 tangent, 9 equal length, 9 horizontal, 8 collinear, 1 coincident, 1 midpoint, 26 other
  measures "d46" distance of L7.start L7.end
  measures "d47" diameter of A0
  measures "d52" distance between parallel lines of L10 L8
  measures "d53" distance between parallel lines of L1 L7
  measures "d54" distance of L19.start L19.end
  measures "d55" diameter of A6
  measures "d56" distance between parallel lines of L12 L21
  measures "d60" distance between parallel lines of L11 L25
  measures "d70" distance between parallel lines of L15 L44
  measures "d71" distance between parallel lines of L20 L46
  measures "d74" distance of L7.start L52.start
extrude "押し出し2" cut sketch "スケッチ7" against normal through all contours L0 L2 L46 A21 A25 L50 L58 A30 A47 L91 L103 A56 A73 L136 L148 A82 L3 L4 A102 L185 L123 A66 A76 L140 L78 A40 A50 L95 L48 A23 A19 L44 | L44 A19 L4 | L2 A21 L46 | A23 L48 L4 | L4 L95 A50 | A40 L78 L4 | L2 L50 A25 | L4 L140 A76 | A66 L123 L4 | L2 A30 L58 | L4 L185 A102 | L2 L91 A47 | A82 L148 L2 | L2 A56 L103 | L136 A73 L2 | L13 A1 L14 A2 L15 A0 | L18 A5 L17 A4 L16 A3 | L22 A7 L23 A8 L24 A6 | L34 A11 L33 A10 L32 A9 | L35 A13 L36 A14 L37 A12 | L43 A17 L41 A16 L42 A15 | L94 A49 L54 A27 L55 A26 | L56 A29 L67 A32 L83 A28 | L61 A33 L65 A35 L63 A34 | L68 A37 L72 A38 L70 A36 | L79 A42 L80 A43 L81 A39 | A44 L89 A46 L87 A45 L85 | L139 A75 L99 A53 L100 A52 | L101 A55 L112 A58 L128 A54 | L106 A59 L110 A61 L108 A60 | L113 A63 L117 A64 L115 A62 | L124 A68 L125 A69 L126 A65 | A70 L134 A72 L132 A71 L130 | L184 A101 L144 A79 L145 A78 | L146 A81 L157 A84 L173 A80 | L151 A85 L155 A87 L153 A86 | L158 A89 L162 A90 L160 A88 | L169 A94 L170 A95 L171 A91 | A96 L179 A98 L177 A97 L175 | L229 A127 L189 A105 L190 A104 | L191 A107 L202 A110 L218 A106 | L196 A111 L200 A113 L198 A112 | L203 A115 L207 A116 L205 A114 | L214 A120 L215 A121 L216 A117 | A122 L224 A124 L222 A123 L220
fillet "フィレット1" radius 1.5 16 edges at (0.75, 81, -2) (0.75, 64.5, -18.5) (0.75, 55.5, -18.5) (0.75, 72, -2) (0.75, 63, -2) (0.75, 54, -2) (0.75, 37.5, -18.5) (0.75, 46.5, -18.5) (-38.75, 46.5, -18.5) (-38.75, 37.5, -18.5) (-38.75, 54, -2) (-38.75, 63, -2) (-38.75, 55.5, -18.5) (-38.75, 64.5, -18.5) (-38.75, 81, -2) (-38.75, 72, -2)
sketch "スケッチ9" plane through (1.5, 0, 0) normal (1, 0, 0) x (0, 0, -1)
  circle A0 centre (17.5, 16) radius 0.8 projected
  circle A1 centre (17.5, 11) radius 0.8 projected
  point P0 (0, 0)
extrude "押し出し3" cut sketch "スケッチ9" against normal through all
sketch "スケッチ10" plane through (-1.5, 0, -25) normal (0, 0, -1) x (-1, 0, 0)
  line L0 (-1.5, 4.9999) -> (-3, 4.9999) projected
  line L1 (-3, 4.9999) -> (38, 4.9999)
  line L2 (38, 4.9999) -> (38, 0)
  line L3 (38, 0) -> (-3, 0)
  line L4 (-3, 0) -> (-3, 4.9999)
  line L5 (35, 0) -> (0, 0) projected
  line L6 (38, 85) -> (38, 4.5826) projected
  point P0 (-1.5, 0)
  point P1 (-1.5, 4.9999)
  constraints: 8 end point, 2 collinear, 2 parallel, 1 horizontal, 1 perpendicular
extrude "押し出し4" cut sketch "スケッチ10" against normal through all
sketch "スケッチ11" plane through (1.5, 0, 0) normal (1, 0, 0) x (0, 0, -1)
  line L0 (0, 97.1421) -> (25, 72.1421)
  line L1 (25, 85) -> (25, 4.9999) projected
  line L2 (4.5607, 78.4393) -> (18.0607, 64.9393) projected
  line L3 (0, 41) -> (0, 85) projected
  line L4 (9.1421, 88) -> (0, 88)
  line L5 (0, 88) -> (-6.0622, 84.5)
  line L6 (-6.0622, 84.5) -> (-6.0622, 64.5)
  line L7 (7.5, 41) -> (0, 41) projected
  line L8 (-6.0622, 64.5) -> (0, 64.5)
  line L9 (0, 85) -> (22, 85) projected
  line L10 (25, 85) -> (22, 85) projected
  point P0 (0, 0)
  point P1 (12.1421, 85)
  dimension "d95" = 10
  dimension "d96" = 23.5
  dimension "d97" = 30
  dimension "d98" = 20
  dimension "d100" = 3
  constraints: 10 end point, 5 point on line, 1 horizontal, 1 parallel, 1 perpendicular, 1 vertical
  measures "d95" distance between parallel lines of L0 L2
  measures "d96" distance from line of L6.end L7
  measures "d97" angle of L4 L5
  measures "d98" distance of L5.end L6.end
  measures "d100" distance between parallel lines of L9 L4
sheet face with bend "面2" sketch "スケッチ11" thickness 1.5 toward (-1, 0, 0) bend radius 1.5 relief straight relief width 1.5 relief depth 0.75 contours L0 L9 L3 L8 L6 L5 L4
bend "曲げ3"
extrude "押し出し5" cut sketch "スケッチ11" against normal through all contours L9 L10 L1 L0
sketch "スケッチ12" plane through (-39.5, 41, 0) normal (-1, 0, 0) x (0, 0, 1)
  circle A0 centre (-17.5, -25) radius 0.8
  circle A1 centre (-17.5, -30) radius 0.8
  line L0 (-9.1421, 47) -> (-22, 34.1421)
  line L1 (-22, 34.1421) -> (-22, -36.0001)
  line L2 (-22, -36.0001) -> (-20.0347, -36.0001)
  line L3 (-15, -30) -> (-20.0347, -36.0001)
  line L4 (-15, -12.9904) -> (-15, -30)
  line L5 (-7.5, 0) -> (-15, -12.9904)
  line L6 (0, 0) -> (-7.5, 0)
  line L7 (0, 23.5) -> (0, 0)
  line L8 (6.0622, 23.5) -> (0, 23.5)
  line L9 (6.0622, 43.5) -> (6.0622, 23.5)
  line L10 (0, 47) -> (6.0622, 43.5)
  line L11 (-9.1421, 47) -> (0, 47)
  line L12 (-2.4393, 30.5607) -> (-15.9393, 17.0607)
  arc A2 (-18.5, 18.1213) -> (-15.9393, 17.0607) centre (-17, 18.1213) ccw
  line L13 (-18.5, 18.1213) -> (-18.5, 22.8787)
  arc A3 (-18.0607, 23.9393) -> (-18.5, 22.8787) centre (-17, 22.8787) ccw
  line L14 (-18.0607, 23.9393) -> (-4.5607, 37.4393)
  arc A4 (-2, 36.3787) -> (-4.5607, 37.4393) centre (-3.5, 36.3787) ccw
  line L15 (-2, 36.3787) -> (-2, 31.6213)
  arc A5 (-2.4393, 30.5607) -> (-2, 31.6213) centre (-3.5, 31.6213) ccw
  line L16 (-2.4393, 12.5607) -> (-15.9393, -0.9393)
  arc A6 (-18.5, 0.1213) -> (-15.9393, -0.9393) centre (-17, 0.1213) ccw
  line L17 (-18.5, 0.1213) -> (-18.5, 4.8787)
  arc A7 (-18.0607, 5.9393) -> (-18.5, 4.8787) centre (-17, 4.8787) ccw
  line L18 (-18.0607, 5.9393) -> (-4.5607, 19.4393)
  arc A8 (-2, 18.3787) -> (-4.5607, 19.4393) centre (-3.5, 18.3787) ccw
  line L19 (-2, 18.3787) -> (-2, 13.6213)
  arc A9 (-2.4393, 12.5607) -> (-2, 13.6213) centre (-3.5, 13.6213) ccw
  line L20 (-12.1421, 44) -> (-22, 34.1421)
  line L21 (-22, 34.1421) -> (-22, -36.0001)
  line L22 (-22, -36.0001) -> (-20.0347, -36.0001)
  line L23 (-20.0347, -36.0001) -> (-15, -30)
  line L24 (-15, -30) -> (-15, -12.9904)
  line L25 (-15, -12.9904) -> (-7.5, 0)
  line L26 (-7.5, 0) -> (0, 0)
  line L27 (0, 44) -> (0, 0)
  line L28 (-12.1421, 44) -> (0, 44)
  circle A10 centre (-17.5, -25) radius 0.8
  circle A11 centre (-17.5, -30) radius 0.8
  line L29 (-2, 18.3787) -> (-2, 13.6213)
  arc A12 (-2.4393, 12.5607) -> (-2, 13.6213) centre (-3.5, 13.6213) ccw
  line L30 (-2.4393, 12.5607) -> (-15.9393, -0.9393)
  arc A13 (-18.5, 0.1213) -> (-15.9393, -0.9393) centre (-17, 0.1213) ccw
  line L31 (-18.5, 0.1213) -> (-18.5, 4.8787)
  arc A14 (-18.0607, 5.9393) -> (-18.5, 4.8787) centre (-17, 4.8787) ccw
  line L32 (-18.0607, 5.9393) -> (-4.5607, 19.4393)
  arc A15 (-2, 18.3787) -> (-4.5607, 19.4393) centre (-3.5, 18.3787) ccw
  line L33 (-18.5, 18.1213) -> (-18.5, 22.8787)
  arc A16 (-18.0607, 23.9393) -> (-18.5, 22.8787) centre (-17, 22.8787) ccw
  line L34 (-18.0607, 23.9393) -> (-4.5607, 37.4393)
  arc A17 (-2, 36.3787) -> (-4.5607, 37.4393) centre (-3.5, 36.3787) ccw
  line L35 (-2, 36.3787) -> (-2, 31.6213)
  arc A18 (-2.4393, 30.5607) -> (-2, 31.6213) centre (-3.5, 31.6213) ccw
  line L36 (-2.4393, 30.5607) -> (-15.9393, 17.0607)
  arc A19 (-18.5, 18.1213) -> (-15.9393, 17.0607) centre (-17, 18.1213) ccw
  point P0 (0, -41)
  point P1 (0, 23.5)
sheet face with bend "面3" sketch "スケッチ12" thickness 1.5 toward (1, 0, 0) bend radius 1.5 relief straight relief width 1.5 relief depth 0.75 contours L11 L10 L9 L8 L27 L28 L0
bend "曲げ4"
sketch "スケッチ13" plane through (-39.5, 11, -15) normal (-1, 0, 0) x (0, 0, 1)
  point P0 (15, -11)
sketch "スケッチ14" plane through (-39.5, 11, -15) normal (-1, 0, 0) x (0, 0, 1)
  circle A0 centre (7.8579, 75) radius 0.8 projected
  circle A1 centre (13, 75) radius 0.8 projected
  circle A2 centre (18.3301, 72.7679) radius 0.8 projected
  point P0 (15, -11)
extrude "押し出し6" cut sketch "スケッチ14" against normal through all
sketch "スケッチ15" plane through (1.5, 0, 0) normal (1, 0, 0) x (0, 0, -1)
  circle A0 centre (-4.0622, 77.5) radius 0.8 projected
  spline S0 degree 3 poles (-4.0622, 73.3) (-4.1628, 73.3) (-4.2701, 73.2798) (-4.4672, 73.1981) (-4.5571, 73.1365) (-4.7005, 72.9931) (-4.7624, 72.9013) (-4.8432, 72.7034) (-4.8622, 72.5973) (-4.8622, 72.3972) (-4.8413, 72.2898) (-4.7595, 72.0938) (-4.6986, 72.0051) (-4.5597, 71.8662) (-4.4724, 71.805) (-4.2763, 71.7219) (-4.1672, 71.7) (-3.9605, 71.7) (-3.8544, 71.7205) (-3.6627, 71.7992) (-3.5768, 71.8572) (-3.4346, 71.9932) (-3.3705, 72.0834) (-3.2843, 72.2838) (-3.2622, 72.3941) (-3.2622, 72.5976) (-3.2812, 72.704) (-3.3625, 72.9024) (-3.4248, 72.9943) (-3.5685, 73.1374) (-3.6582, 73.1986) (-3.8549, 73.28) (-3.9619, 73.3) (-4.0622, 73.3) knots 0 0 0 0 0.030185 0.030185 0.060371 0.060371 0.091344 0.091344 0.122317 0.122317 0.15503 0.15503 0.187744 0.187744 0.21924 0.21924 0.250737 0.250737 0.281251 0.281251 0.311765 0.311765 0.345449 0.345449 0.379133 0.379133 0.410197 0.410197 0.441261 0.441261 0.471356 0.471356 0.501451 0.501451 0.501451 0.501451 projected
  circle A1 centre (-4.0622, 72.5) radius 0.8 projected
  point P0 (0, 0)
  point P1 (-4.0622, 73.3)
  constraints: 1 vertical alignment
extrude "押し出し7" cut sketch "スケッチ15" against normal through all
fillet "フィレット2" radius 3 4 edges at (0.75, 64.5, 0) (0.75, 64.5, 6.0622) (-38.75, 64.5, 0) (-38.75, 64.5, 6.0622)
equation "\"d18\" = d16"
equation "\"d20\" = Thickness"
equation "\"d45\" = d44"
equation "\"d56\" = d52"
equation "\"d70\" = d52"
equation "\"d71\" = d70"
equation "\"d13\" = Thickness"
equation "\"d22\" = BendReliefWidth"
equation "\"d23\" = BendReliefDepth"
equation "\"d24\" = MinimumRemnant"
equation "\"d25\" = TransitionRadius"
equation "\"d28\" = BendRadius"
equation "\"d29\" = CornerReliefSize"
equation "\"d30\" = GapSize"
equation "\"d31\" = JacobiRadiusSize"
equation "\"d32\" = BendReliefWidth"
equation "\"d33\" = BendReliefDepth"
equation "\"d34\" = MinimumRemnant"
equation "\"d35\" = TransitionRadius"
equation "\"d38\" = BendRadius"
equation "\"d39\" = CornerReliefSize"
equation "\"d40\" = GapSize"
equation "\"d41\" = JacobiRadiusSize"
equation "\"BendRadius\" = Thickness"
equation "\"BendReliefWidth\" = Thickness"
equation "\"BendReliefDepth\" = 0.5 * Thickness"
equation "\"CornerReliefSize\" = 4 * Thickness"
equation "\"MinimumRemnant\" = 2 * Thickness"
equation "\"TransitionRadius\" = BendRadius"
equation "\"JacobiRadiusSize\" = BendRadius"
equation "\"GapSize\" = Thickness"
equation "\"Thickness\" = 1.5"
